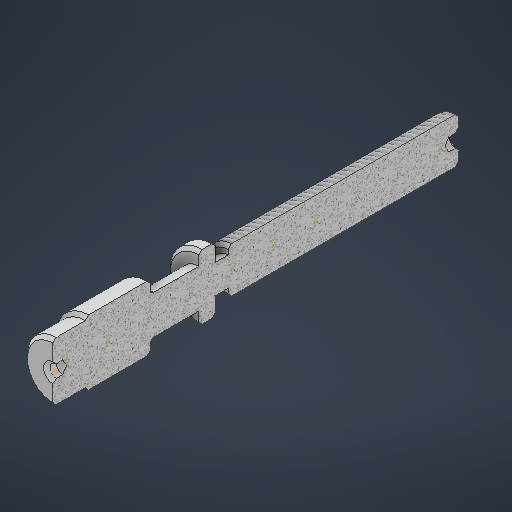
# Autodesk Inventor part: b7
Saved by Autodesk Inventor 2025.4 (Build 294407000, 407)
## iProperties
Created: 2026-05-15
Part Number: b7
Material: Generic
Document SubType Name: Modeling
Designer: VuQuan
Density: 1 g/cm^3
Appearance: Default
Author: VuQuan
Autodesk Inventor part; units mm, degrees
ref_plane "YZ Plane" through (0, 0, 0) normal (1, 0, 0) x (0, 1, 0)
ref_plane "XZ Plane" through (0, 0, 0) normal (0, 1, 0) x (-1, 0, 0)
ref_plane "XY Plane" through (0, 0, 0) normal (0, 0, 1) x (1, 0, 0)
sketch "Sketch1" plane through (0, 0, 0) normal (1, 0, 0) x (0, 1, 0)
  line L0 (0, 0) -> (9, 0)
  line L1 (9, 0) -> (9, -10)
  line L2 (9, -10) -> (10, -10)
  line L3 (10, -10) -> (10, -30)
  line L4 (10, -30) -> (6, -30)
  line L5 (6, -30) -> (6, -45)
  line L6 (6, -45) -> (10, -45)
  line L7 (10, -45) -> (10, -50)
  line L8 (0, 0) -> (0, -125)
  line L9 (10, -50) -> (4.5, -50)
  line L10 (4.5, -50) -> (4.5, -54)
  line L11 (4.5, -54) -> (7, -54)
  line L12 (7, -54) -> (7, -125)
  line L13 (7, -125) -> (0, -125)
  dimension "d1" = 18
  dimension "d2" = 20
  dimension "d3" = 12
  dimension "d4" = 20
  dimension "d5" = 9
  dimension "d6" = 14
  dimension "d7" = 20
  dimension "d8" = 15
  dimension "d9" = 4
  dimension "d10" = 5
  dimension "d11" = 71
  dimension "d12" = 125
  constraints: 28 end point, 11 perpendicular, 2 horizontal, 1 vertical
  measures "d1" diameter of L1 L8
  measures "d2" diameter of L3 L8
  measures "d3" diameter of L5 L8
  measures "d4" diameter of L7 L8
  measures "d5" diameter of L10 L8
  measures "d6" diameter of L12 L8
  measures "d7" distance of L2.end L3.end
  measures "d8" distance between parallel lines of L6 L4
  measures "d9" distance between parallel lines of L11 L9
  measures "d10" distance between parallel lines of L9 L6
  measures "d11" distance between parallel lines of L13 L11
  measures "d12" distance between parallel lines of L13 L0
revolve "Revolution1" add sketch "Sketch1" angle 360 about axis through (0, 0, 0) along (0, 0, -1)
thread "Thread1" size "M14x2" class "6g" standard "ANSI Metric M Profile" full length
hole "Hole1" at (0, 0, 0) direction (0, 0, -1) diameter 4 depth 3 tip angle 118
sketch "Sketch2" plane through (0, 0, -125) normal (0, 0, -1) x (-1, 0, 0)
  point P0 (0, 0)
  point P1 (0, 0)
  constraints: 1 coincident
hole "Hole2" at (0, 0, -125) direction (0, 0, 1) diameter 4 depth 3 tip angle 118
chamfer "Chamfer1" distance 1 angle 45 9 edges at (0, -9, 0) (0, 2, 0) (0, -10, -10) (0, -10, -45) (0, -10, -50) (0, -7, -54) (0, -7, -125) (0, -2, -125) (0, -10, -30)
fillet "Fillet1" radius 1 1 edges at (0, -6, -30)
body "Solid1"
